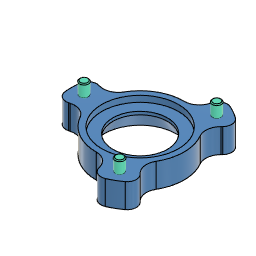
PadGlueJig_Parametric (Autodesk Fusion 360 design; units mm, degrees)
Autodesk Fusion 360 part; units mm, degrees
note: some values were not read from the file. Set by a fixed rule: which sketch regions a step uses.
sketch "Sketch1" plane through (0, 0, 0) normal (0, 0, 1) x (1, 0, 0)
  circle A0 centre (0, 0) radius 22.5
  circle A1 centre (0, 0) radius 9
  dimension "d1" = 45
  dimension "d2" = 18
  constraint coincident A0.centre A1.centre
  measures "d1" diameter of A0
  measures "d2" diameter of A1
extrude "Extrude1" add sketch "Sketch1" along normal blind 8 makes body 1
sketch "Sketch2" plane through (0, 0, 8) normal (0, 0, 1) x (-1, 0, 0)
  circle A0 centre (0, 0) radius 9
  circle A1 centre (0, 0) radius 22.5
  circle A2 centre (18.5, 0) radius 1.35
  circle A3 centre (0, 0) radius 14.5
  line L0 (0, 0) -> (21.7333, -5.8234)
  line L1 (0, 0) -> (-5.8234, -21.7333)
  line L2 (0, 0) -> (18.5, 0) construction
  dimension "d5" = 2.7
  dimension "d6" = 18.5
  dimension "d7" = 90
  dimension "d8" = 15
  dimension "d9" = 29
  constraint horizontal A0.centre A2.centre
  constraint coincident A0.centre A1.centre
  constraint coincident A1 L0.end
  constraint coincident A1 L1.end
  constraint coincident A2.centre L2.end
  measures "d5" diameter of A2
  measures "d6" distance of A0.centre A2.centre
  measures "d7" angle of L0 L1
  measures "d8" angle of L0 L2
  measures "d9" diameter of A3
extrude "Extrude2" cut sketch "Sketch2" against normal blind 14 contours A1 A3 L0 L1 | A2 picked at (18.8075, -6.1445) bodies 1
sketch "Sketch4" plane through (0, 0, 0) normal (0, 0, 1) x (-1, 0, 0)
  line L0 (12.0741, -3.2352) -> (19.3185, -5.1764)
  line L1 (-5.1764, -19.3185) -> (-3.2352, -12.0741)
  arc A0 (-3.2352, -12.0741) -> (12.0741, -3.2352) centre (0, 0) ccw
  circle A1 centre (18.5, 0) radius 3
  line L2 (21.7333, -5.8234) -> (14.0059, -3.7529)
  line L3 (-3.7529, -14.0059) -> (-5.8234, -21.7333)
  arc A2 (21.7333, -5.8234) -> (-5.8234, -21.7333) centre (0, 0) ccw
  circle A3 centre (18.5, 0) radius 1.35
  arc A4 (-3.7529, -14.0059) -> (14.0059, -3.7529) centre (0, 0) ccw
  circle A5 centre (0, 0) radius 9
  dimension "d20" = 6
  constraint concentric A1 A3
  measures "d20" diameter of A1
extrude "Extrude3" cut sketch "Sketch4" along normal blind 4 contours A1 | A3 bodies 1
sketch "Sketch6" plane through (0, 0, 4) normal (0, 0, -1) x (1, 0, 0)
  circle A0 centre (-18.5, 0) radius 1.35
  circle A1 centre (-18.5, 0) radius 1.35
  circle A2 centre (-18.5, 0) radius 3
  constraint equal A0 A1
  constraint concentric A0 A1
extrude "Extrude5" add sketch "Sketch6" against normal blind 0.25 contours A0 A1 bodies 1
pattern_circular "C-Pattern1" count 3 over 360 about axis through (0, 0, 1.75) along (0, 0, 1) of "Extrude2", "Extrude3", "Extrude5"
fillet "Fillet1" radius 5 6 edges at (-14.0059, -3.7529, 4) (3.7529, -14.0059, 4) (10.253, -10.253, 4) (10.253, 10.253, 4) (3.7529, 14.0059, 4) (-14.0059, 3.7529, 4) on bodies 1
fillet "Fillet2" radius 3 6 edges at (5.8234, 21.7333, 4) (15.9099, 15.9099, 4) (-21.7333, 5.8234, 4) (-21.7333, -5.8234, 4) (5.8234, -21.7333, 4) (15.9099, -15.9099, 4) on bodies 1
chamfer "Chamfer1" distance 5 angle 30 1 edges at (-8.3909, 3.2545, 0) measured on face at (8.9888, -0.4486, 5.3333) on bodies 1
sketch "Sketch5" plane through (0, 0, 8) normal (0, 0, 1) x (-1, 0, 0)
  arc A0 (-13.2728, 18.1682) -> (-13.6244, 13.6244) centre (-11.5031, 15.7457) ccw
  arc A1 (-12.5393, 7.2813) -> (-13.3276, 13.3276) centre (-16.8631, 9.7921) ccw
  arc A2 (18.6113, -4.9869) -> (22.3705, -2.4105) centre (19.3878, -2.0891) ccw
  arc A3 (-13.2728, -18.1682) -> (-9.0977, -20.5787) centre (0, 0) ccw
  arc A4 (22.3705, 2.4105) -> (18.6113, 4.9869) centre (19.3878, 2.0891) ccw
  arc A5 (12.5754, 7.2187) -> (18.2058, 4.8782) centre (16.9117, 9.7079) ccw
  arc A6 (-4.9869, 18.6113) -> (-9.0977, 20.5787) centre (-7.8847, 17.8349) ccw
  arc A7 (-9.0977, 20.5787) -> (-13.2728, 18.1682) centre (0, 0) ccw
  circle A8 centre (18.5, 0) radius 1.35
  circle A9 centre (-9.25, 16.0215) radius 1.35
  circle A10 centre (0, 0) radius 12.65
  line L0 (18.2058, -4.8782) -> (18.6113, -4.9869)
  line L1 (18.6113, 4.9869) -> (18.2058, 4.8782)
  line L2 (-4.8782, 18.2058) -> (-4.9869, 18.6113)
  line L3 (-13.6244, 13.6244) -> (-13.3276, 13.3276)
  arc A11 (-13.3276, -13.3276) -> (-12.5393, -7.2813) centre (-16.8631, -9.7921) ccw
  line L4 (-13.3276, -13.3276) -> (-13.6244, -13.6244)
  arc A12 (-13.6244, -13.6244) -> (-13.2728, -18.1682) centre (-11.5031, -15.7457) ccw
  arc A13 (-9.0977, -20.5787) -> (-4.9869, -18.6113) centre (-7.8847, -17.8349) ccw
  line L5 (-4.9869, -18.6113) -> (-4.8782, -18.2058)
  arc A14 (-0.0361, -14.5) -> (-4.8782, -18.2058) centre (-0.0486, -19.4999) ccw
  arc A15 (-0.0361, -14.5) -> (12.5754, -7.2187) centre (0, 0) ccw
  arc A16 (18.2058, -4.8782) -> (12.5754, -7.2187) centre (16.9117, -9.7079) ccw
  arc A17 (12.5754, 7.2187) -> (-0.0361, 14.5) centre (0, 0) ccw
  arc A18 (-4.8782, 18.2058) -> (-0.0361, 14.5) centre (-0.0486, 19.4999) ccw
  arc A19 (-12.5393, 7.2813) -> (-12.5393, -7.2813) centre (0, 0) ccw
  circle A20 centre (-9.25, -16.0215) radius 1.35
  arc A21 (22.3705, -2.4105) -> (22.3705, 2.4105) centre (0, 0) ccw
  circle A22 centre (0, 0) radius 9
  dimension "d23" = 25.3
  constraint coincident A3.centre A7.centre
  measures "d23" diameter of A10
extrude "Extrude4" cut sketch "Sketch5" against normal blind 2 contours A10 bodies 1
sketch "Sketch1 (2)" plane through (0, 0, 0) normal (0, 0, 1) x (1, 0, 0) in component "Screw1_M3 v1"
  circle A0 centre (0, 0) radius 1.5
  dimension "d760" = 3
  constraint coincident A0.centre origin
  measures "d760" diameter of A0
extrude "Extrude1'" add sketch "Sketch1 (2)" against normal blind 10 separate body makes body 2 in component "Screw1_M3 v1"
sketch "Sketch2 (2)" plane through (0, 0, -10) normal (0, 0, -1) x (1, 0, 0) in component "Screw1_M3 v1"
  circle A0 centre (0, 0) radius 1.5
  circle A1 centre (0, 0) radius 2.75
  dimension "d763" = 5.5
  constraint concentric A0 A1
  measures "d763" diameter of A1
extrude "Extrude2'" add sketch "Sketch2 (2)" along normal blind 2.75 contours A0 | A1 bodies 2 in component "Screw1_M3 v1"
sketch "Sketch3" plane through (0, 0, -12.75) normal (0, 0, -1) x (1, 0, 0) in component "Screw1_M3 v1"
  circle A0 centre (0, 0) radius 2.75
  line L0 (1.25, 0.7217) -> (0, 1.4434)
  line L1 (0, 1.4434) -> (-1.25, 0.7217)
  line L2 (-1.25, 0.7217) -> (-1.25, -0.7217)
  line L3 (-1.25, -0.7217) -> (0, -1.4434)
  line L4 (0, -1.4434) -> (1.25, -0.7217)
  line L5 (1.25, -0.7217) -> (1.25, 0.7217)
  dimension "d766" = 2.5
  constraint coincident A0.centre origin
  measures "d766" distance of L2 L5
extrude "Extrude3'" cut sketch "Sketch3" against normal blind 2 contours L0 L1 L2 L3 L4 L5 bodies 2 in component "Screw1_M3 v1"
fillet "Fillet1'" radius 0.25 1 edges at (-1.3985, 0.5424, -10) on bodies 2 in component "Screw1_M3 v1"
chamfer "Chamfer1'" distance 0.1 angle 45 2 edges at (-2.5639, 0.9944, -12.75) (-2.5639, 0.9944, -10) on bodies 2 in component "Screw1_M3 v1"
chamfer "Chamfer2" distance 0.3 angle 45 1 edges at (-1.3985, -0.5424, 0) on bodies 2 in component "Screw1_M3 v1"
component "Screw1_M3 v1" placed x (-0.877067, -0.480368, 0) y (0.480368, -0.877067, 0) z (0, 0, 1) at (9.25, -16.0215, 13.025)
component "Screw1_M3 v1" placed x (0.866025, 0.5, 0) y (-0.5, 0.866025, 0) z (0, 0, 1) at (9.25, 16.0215, 13.025)
component "Screw1_M3 v1" placed x (0.877067, 0.480368, 0) y (-0.480368, 0.877067, 0) z (0, 0, 1) at (-18.5, 0, 13.025)
equation "d1 = D + 20 mm"
equation "d2 = D - 7 mm"
equation "d6 = D / 2 + 6 mm"
equation "d9 = D + 4 mm"
equation "d23 = D + 0.3 mm"
equation "D = 25 mm" comment "Pad Diameter"
named bodies: "PadGlueRig", "PadGlueRig (1)"
